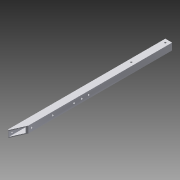
# Autodesk Inventor part: pickup arm 1x1
Saved by Autodesk Inventor 2015 (Build 190159000, 159)
## iProperties
Created: 2015-01-27
Part Number: pickup arm 1x1
Material: Aluminum 6061
Document SubType Name: Modeling
Designer: Admin
Density: 2.7 g/cm^3
Appearance: Aluminum - Flat
Author: Admin
Autodesk Inventor part; units mm, degrees
ref_plane "YZ Plane" through (0, 0, 0) normal (1, 0, 0) x (0, 1, 0)
ref_plane "XZ Plane" through (0, 0, 0) normal (0, 1, 0) x (-1, 0, 0)
ref_plane "XY Plane" through (0, 0, 0) normal (0, 0, 1) x (1, 0, 0)
sketch "Sketch1" plane through (0, 0, 0) normal (0, 0, 1) x (1, 0, 0)
  line L0 (0, 0) -> (25.4, 0)
  line L1 (25.4, 0) -> (25.4, 25.4)
  line L2 (25.4, 25.4) -> (0, 25.4)
  line L3 (0, 25.4) -> (0, 0)
  line L4 (3.175, 3.175) -> (22.225, 3.175)
  line L5 (22.225, 3.175) -> (22.225, 22.225)
  line L6 (22.225, 22.225) -> (3.175, 22.225)
  line L7 (3.175, 22.225) -> (3.175, 3.175)
  dimension "d0" = 25.4
  dimension "d1" = 25.4
  dimension "d2" = 19.05
  dimension "d3" = 19.05
  dimension "d4" = 3.175
  dimension "d5" = 3.175
  constraints: 16 end point, 4 parallel, 2 horizontal, 2 perpendicular
  measures "d0" distance of L2.end L1.end
  measures "d1" distance of L1.end L0.end
  measures "d2" distance of L6.end L5.end
  measures "d3" distance of L5.end L4.end
  measures "d4" distance between parallel lines of L0 L4
  measures "d5" distance between parallel lines of L3 L7
extrude "Extrusion1" add sketch "Sketch1" along normal blind 587.375
sketch "Sketch2" plane through (0, 25.4, 0) normal (0, 1, 0) x (1, 0, 0)
  line L0 (25.4, 0) -> (0, 0) projected
  line L1 (0, 0) -> (0, -587.375) projected
  point P0 (12.7, -12.7)
  point P1 (12.7, -139.7)
  dimension "d8" = 12.7
  dimension "d9" = 12.7
  dimension "d10" = 12.7
  dimension "d11" = 139.7
  measures "d8" distance from line of L0 point (12.7, -12.7)
  measures "d9" distance from line of L1 point (12.7, -12.7)
  measures "d10" distance from line of L1 point (12.7, -139.7)
  measures "d11" distance from line of L0 point (12.7, -139.7)
hole "Hole1" at (12.7, 25.4, 12.7) at (12.7, 25.4, 139.7) direction (0, -1, 0) diameter 6.35 end through all
sketch "Sketch3" plane through (25.4, 0, 0) normal (1, 0, 0) x (0, 0, -1)
  line L0 (-587.375, 0) -> (-587.375, 25.4) projected
  line L1 (0, 0) -> (-587.375, 0) projected
  point P0 (-574.675, 12.7)
  point P1 (-549.275, 12.7)
  point P2 (-336.55, 12.7)
  point P3 (-311.15, 12.7)
  dimension "d19" = 12.7
  dimension "d20" = 12.7
  dimension "d21" = 12.7
  dimension "d22" = 25.4
  dimension "d23" = 212.725
  dimension "d24" = 25.4
  dimension "d25" = 12.7
  dimension "d26" = 12.7
  measures "d19" distance from line of L0 point (-574.675, 12.7)
  measures "d20" distance from line of L1 point (-574.675, 12.7)
  measures "d21" distance from line of L1 point (-549.275, 12.7)
  measures "d22" distance of point (-574.675, 12.7) point (-549.275, 12.7)
  measures "d23" distance of point (-336.55, 12.7) point (-549.275, 12.7)
  measures "d24" distance of point (-336.55, 12.7) point (-311.15, 12.7)
  measures "d25" distance from line of L1 point (-311.15, 12.7)
  measures "d26" distance from line of L1 point (-336.55, 12.7)
hole "Hole2" at (25.4, 12.7, 574.675) at (25.4, 12.7, 549.275) at (25.4, 12.7, 336.55) at (25.4, 12.7, 311.15) direction (-1, 0, 0) diameter 6.35 end through all
sketch "Sketch6" plane through (0, 25.4, 0) normal (0, 1, 0) x (1, 0, 0)
  circle A0 centre (12.7, -12.7) radius 3.175 projected
  circle A1 centre (12.7, -139.7) radius 3.175 projected
  line L0 (25.4, 0) -> (0, 0) projected
  line L1 (0, 0) -> (0, -587.375) projected
  line L2 (25.4, -587.375) -> (0, -587.375) projected
  line L3 (25.4, 0) -> (25.4, -587.375) projected
  line L4 (25.4, -587.375) -> (3.175, -587.375)
  line L5 (0, -587.375) -> (25.4, -587.375) projected
  line L6 (25.4, -587.375) -> (25.4, -536.575)
  line L7 (25.4, 0) -> (25.4, -587.375) projected
  line L8 (25.4, -536.575) -> (3.175, -587.375)
  dimension "d41" = 22.225
  dimension "d42" = 50.8
  constraints: 6 end point, 1 collinear, 1 point on line
  measures "d41" distance of L2.start L4.end
  measures "d42" distance of L2.start L6.end
extrude "Extrusion4" cut sketch "Sketch6" against normal blind 25.4 contours L3 L2 L8
sketch "Sketch7" plane through (0, 0, 0) normal (-1, 0, 0) x (0, 0, 1)
  line L0 (587.375, 25.4) -> (587.375, 0) projected
  line L1 (0, 25.4) -> (587.375, 25.4) projected
  point P0 (365.125, 12.7)
  point P1 (444.5, 12.7)
  point P2 (523.875, 12.7)
  dimension "d45" = 12.7
  dimension "d46" = 63.5
  dimension "d47" = 12.7
  dimension "d48" = 12.7
  dimension "d49" = 142.875
  dimension "d50" = 222.25
  measures "d45" distance from line of L1 point (523.875, 12.7)
  measures "d46" distance from line of L0 point (523.875, 12.7)
  measures "d47" distance from line of L1 point (444.5, 12.7)
  measures "d48" distance from line of L1 point (365.125, 12.7)
  measures "d49" distance from line of L0 point (444.5, 12.7)
  measures "d50" distance from line of L0 point (365.125, 12.7)
hole "Hole3" at (0, 12.7, 365.125) at (0, 12.7, 444.5) at (0, 12.7, 523.875) direction (1, 0, 0) diameter 6.35 end through all
body "Solid1"
